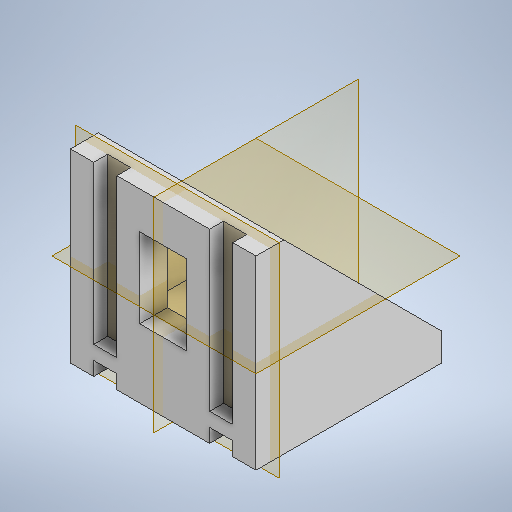
# Autodesk Inventor part: Soporte_2020_0001
Saved by Autodesk Inventor 2025.2 (Build 292293000, 293)
## iProperties
Created: 2025-04-07
Part Number: Soporte_2020_0001
Material: Genérico
Document SubType Name: Modeling
Designer: samre
Density: 1 g/cm^3
Appearance: Valor por defecto
Author: Miguel
Autodesk Inventor part; units mm, degrees
sketch "Boceto1" plane through (0, 0, 0) normal (0, 0, 1) x (1, 0, 0)
  line L0 (10, -10) -> (-10, -10)
  line L1 (-10, -10) -> (-10, 10)
  line L2 (-10, 10) -> (10, 10)
  line L3 (10, 10) -> (10, -10)
  line L4 (10, -10) -> (-10, 10) construction
  line L5 (-10, -10) -> (10, 10) construction
  line L6 (2.55, 6) -> (-2.55, 6) construction
  line L7 (-2.55, 6) -> (2.55, 6)
  line L8 (2.55, 6) -> (2.55, -2.6)
  line L9 (2.55, -2.6) -> (-2.55, -2.6)
  line L10 (-2.55, -2.6) -> (-2.55, 6)
  point P0 (0, 0)
  point P1 (0, 6)
  dimension "d0" = 20
  dimension "d1" = 4
  dimension "d2" = 5.1
  dimension "d3" = 8.6
  constraints: 22 end point, 4 parallel, 3 horizontal, 3 midpoint, 3 perpendicular, 1 vertical alignment
  measures "d0" distance of L1.end L2.end
  measures "d1" distance between parallel lines of L6 L2
  measures "d2" distance of L6.start L6.end
  measures "d3" distance of L6.start L8.end
extrude "Extrusión1" add sketch "Boceto1" along normal mid plane 3
sketch "Boceto2" plane through (0, 0, 1.5) normal (0, 0, 1) x (1, 0, 0)
  line L0 (10, 10) -> (-10, 10) projected
  line L1 (-10, -10) -> (10, -10) projected
  line L2 (-7.5, 10) -> (-5, 10)
  line L3 (-5, 10) -> (-5, -10)
  line L4 (-5, -10) -> (-7.5, -10)
  line L5 (-7.5, -10) -> (-7.5, 10)
  line L6 (5, 10) -> (7.5, 10)
  line L7 (7.5, 10) -> (7.5, -10)
  line L8 (7.5, -10) -> (5, -10)
  line L9 (5, -10) -> (5, 10)
  line L10 (0, -14) -> (0, 14) projected
  point P0 (0, 0)
  point P1 (-5, 10)
  point P2 (5, -10)
  dimension "d6" = 2.5
  dimension "d7" = 5
  constraints: 16 end point, 5 parallel, 4 point on line, 2 horizontal, 2 perpendicular, 2 other
  measures "d6" distance of L3.end L4.end
  measures "d7" distance from line of point (0, 0) L3
extrude "Extrusión2" cut sketch "Boceto2" against normal blind 1.5 contours L7 L1 L9 L0 | L3 L1 L5 L0
sketch "Boceto5" plane through (-10, -10, -1.5) normal (0, -1, 0) x (1, 0, 0)
  line L0 (20, -17) -> (0, -17)
  line L1 (0, -17) -> (0, 3)
  line L2 (0, 3) -> (20, 3)
  line L3 (20, 3) -> (20, -17)
  line L4 (20, -17) -> (0, 3) construction
  line L5 (0, -17) -> (20, 3) construction
  line L6 (12.5, -4.5) -> (7.5, -4.5) construction
  line L7 (7.5, -4.5) -> (12.5, -4.5)
  line L8 (12.5, -4.5) -> (12.5, -13)
  line L9 (12.5, -13) -> (7.5, -13)
  line L10 (7.5, -13) -> (7.5, -4.5)
  point P0 (10, 1.5)
  point P1 (10, -7)
  point P2 (10, -4.5)
  dimension "d12" = 20
  dimension "d14" = 5
  dimension "d15" = 8.5
  dimension "d16" = 4
  constraints: 22 end point, 4 parallel, 3 horizontal, 3 midpoint, 3 perpendicular, 1 coincident, 1 vertical alignment
  measures "d12" distance of L1.end L2.end
  measures "d14" distance of L6.start L6.end
  measures "d15" distance of L6.start L8.end
  measures "d16" distance between parallel lines of L0 L9
extrude "Extrusión3" add sketch "Boceto5" against normal blind 3
sketch "Boceto6" plane through (-10, -10, 1.5) normal (0, -1, 0) x (1, 0, 0)
  line L0 (0, -20) -> (20, -20) projected
  line L1 (15, 0) -> (5, 0) projected
  line L2 (17.5, -20) -> (15, -20)
  line L3 (15, -20) -> (15, 0)
  line L4 (15, 0) -> (17.5, 0)
  line L5 (17.5, 0) -> (17.5, -20)
  line L6 (7.5, -7.5) -> (12.5, -7.5) projected
  line L7 (2.5, 0) -> (5, 0) projected
  line L8 (5, -20) -> (2.5, -20)
  line L9 (2.5, -20) -> (2.5, 0)
  line L10 (2.5, 0) -> (5, 0)
  line L11 (5, 0) -> (5, -20)
  line L12 (10, -24) -> (10, 4) projected
  point P0 (10, -1.5)
  point P1 (10, -7.5)
  point P2 (10, -7.5)
  point P3 (2.5, -20)
  dimension "d19" = 2.5
  dimension "d20" = 5
  constraints: 16 end point, 4 parallel, 4 point on line, 2 horizontal, 2 midpoint, 2 perpendicular, 2 other
  measures "d19" distance of L3.end L4.end
  measures "d20" distance from line of point (10, -7.5) L3
extrude "Extrusión4" cut sketch "Boceto6" against normal blind 1.5 contours L9 L7 L11 L0 | L3 L4 L5 L0
sketch "Boceto7" plane through (10, -10, 1.5) normal (1, 0, 0) x (0, 0, -1)
  line L0 (0, 20) -> (3, 20) projected
  line L1 (20, 0) -> (20, 3) projected
  line L2 (3, 20) -> (20, 3)
  line L3 (20, 3) -> (3, 3)
  line L4 (3, 3) -> (3, 20)
  point P0 (1.5, 10)
  constraints: 6 end point, 2 perpendicular
extrude "Extrusión5" add sketch "Boceto7" against normal blind 1.5
mirror "Simetría1" about plane through (0, 0, 0) normal (1, 0, 0) of "Extrusión5"
